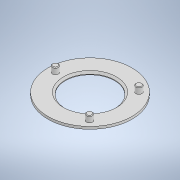
# Autodesk Inventor part: Шапка лидара
Saved by Autodesk Inventor 2020 (Build 240168000, 168)
## iProperties
Created: 2021-08-20
Part Number: Шапка лидара
Material: Типовые
Document SubType Name: Modeling
Designer: Антон
Density: 1 g/cm^3
Appearance: По умолчанию
Author: Антон
Autodesk Inventor part; units mm, degrees
ref_plane "YZ Plane" through (0, 0, 0) normal (1, 0, 0) x (0, 1, 0)
ref_plane "XZ Plane" through (0, 0, 0) normal (0, 1, 0) x (-1, 0, 0)
ref_plane "XY Plane" through (0, 0, 0) normal (0, 0, 1) x (1, 0, 0)
sketch "Эскиз1" plane through (0, 0, 0) normal (0, 1, 0) x (-1, 0, 0)
  circle A0 centre (0, 0) radius 34
  dimension "d0" = 68
  constraints: 1 centre point, 1 coincident
  measures "d0" diameter of A0
extrude "Выдавливание1" add sketch "Эскиз1" along normal blind 2
sketch "Эскиз2" plane through (0, 2, 0) normal (0, 1, 0) x (1, 0, 0)
  circle A0 centre (0, 0) radius 28
  line L0 (19.5959, -20) -> (19.5959, 20)
  line L1 (19.5959, -20) -> (-28, 0)
  line L2 (19.5959, 20) -> (-28, 0)
  circle A1 centre (-28, 0) radius 2.5
  circle A2 centre (19.5959, -20) radius 2.5
  circle A3 centre (19.5959, 20) radius 2.5
  dimension "d3" = 56
  dimension "d4" = 40
  dimension "d5" = 5
  constraints: 6 end point, 4 centre point, 4 coincident, 3 point on circle, 2 equal radius, 1 equal length, 1 vertical
  measures "d3" diameter of A0
  measures "d4" distance of L0.start L0.end
  measures "d5" diameter of A1
extrude "Выдавливание2" add sketch "Эскиз2" along normal blind 5 contours A3 L0 A0 | A0 A3 | A2 A0 | A0 L0 A2 | L2 A3 A0 | L0 A3 L2 | L1 A2 L0 | A0 A2 L1 | A1 L2 A0 | A0 A1 | A1 L1 L2 | A0 L1 A1
chamfer "Фаска1" distance 0.5 angle 45 3 edges at (17.0959, 7, -20) (17.0959, 7, 20) (-30.5, 7, 0)
sketch "Эскиз3" plane through (0, 2, 0) normal (0, 1, 0) x (1, 0, 0)
  circle A0 centre (0, 0) radius 20
  dimension "d11" = 40
  constraints: 1 centre point, 1 coincident
  measures "d11" diameter of A0
extrude "Выдавливание3" cut sketch "Эскиз3" against normal blind 5
chamfer "Фаска2" distance 1.5 angle 45 1 edges at (-20, 2, 0)
